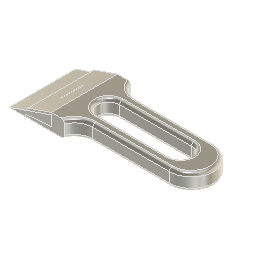
Скребок (Autodesk Fusion 360 design; units mm, degrees)
Autodesk Fusion 360 part; units mm, degrees
note: some values were not read from the file. Set by a fixed rule: which sketch regions a step uses.
sketch "Sketch1" plane through (0, 0, 0) normal (0, 0, 1) x (1, 0, 0)
  line L0 (60, -30) -> (-60, -30)
  line L1 (-60, -30) -> (-60, 30)
  line L2 (-60, 30) -> (60, 30)
  line L3 (60, -30) -> (-60, 30) construction
  line L4 (-60, -30) -> (60, 30) construction
  line L5 (-25, -20) -> (-25, 20)
  line L6 (-25, 20) -> (60, 20)
  line L7 (-25, -20) -> (60, -20)
  line L8 (-25, -20) -> (-25, -30)
  line L9 (-25, 20) -> (-25, 30)
  line L10 (-25, 10) -> (50, 10)
  line L11 (-25, -10) -> (50, -10)
  arc A0 (50, -10) -> (50, 10) centre (50, 0) ccw
  arc A1 (60, -20) -> (60, 20) centre (60, 0) ccw
  line L12 (60, 30) -> (60, 20)
  line L13 (60, -20) -> (60, -30)
  constraint horizontal L0
  constraint perpendicular L0 L1
  constraint parallel L0 L2
  constraint parallel L1 L12
  constraint coincident L3 origin
  constraint coincident L4 origin
  constraint vertical L5
  constraint perpendicular L6 L12
  constraint coincident L7.end L12
  constraint perpendicular L7 L12
  constraint perpendicular L7 L8
  constraint coincident L2 L9.end
  constraint perpendicular L2 L9
  constraint tangent L10 A0
  constraint collinear L12 L13
extrude "Extrude1" add sketch "Sketch1" along normal blind 15 contours L0 L1 L2 L5 L8 L9 | L5 L6 L7 L10 L11 A0 A1 makes body 1
sketch "Sketch2" plane through (0, -30, 0) normal (0, -1, 0) x (1, 0, 0)
  line L0 (-60, 0) -> (-25, 0)
  line L1 (-25, 0) -> (-25, 15)
  line L2 (-25, 15) -> (-60, 15)
  line L3 (-60, 15) -> (-60, 0)
  line L4 (-75.0675, 0) -> (-36.9699, 13.0336)
  line L5 (-75.0675, 0) -> (-60, 0)
  line L6 (-60, 0) -> (-60, 1.9989)
  line L7 (-60, 1.9989) -> (-36.9699, 4.0017)
  line L8 (-36.9699, 4.0017) -> (-36.9699, 13.0336)
  line L9 (-48.7521, 10.4269) -> (-47.477, 10.8632)
  line L10 (-47.477, 10.8632) -> (-47.477, 9.439)
  line L11 (-49.9999, 8.5759) -> (-48.7521, 10.4269)
  point P0 (-50.0767, 9.9738)
  constraint coincident L0.start L3.end
  constraint perpendicular L3 L5
  constraint coincident L3 L6.end
  constraint parallel L3 L8
  constraint parallel L4 L9
  constraint coincident L4 L10.end
  constraint perpendicular L0 L10
  constraint coincident P0 L9
  constraint coincident L4 L11.start
extrude "Extrude2" cut sketch "Sketch2" against normal blind 79 contours L3 L4 L5 L6 | L3 L4 L7 L8 bodies 1
sketch "Sketch3" plane through (0, -30, 0) normal (0, -1, 0) x (1, 0, 0)
  line L0 (-60, 5.1547) -> (-36.9699, 13.0336)
  line L1 (-36.9699, 13.0336) -> (-36.9699, 4.0017)
  line L2 (-36.9699, 4.0017) -> (-60, 1.9989)
  line L3 (-60, 1.9989) -> (-60, 0)
  line L4 (-60, 0) -> (-25, 0)
  line L5 (-25, 0) -> (-25, 15)
  line L6 (-25, 15) -> (-60, 15)
  line L7 (-37, 15) -> (-60, 15)
  line L8 (-60, 5.1547) -> (-60, 7.1547)
  line L9 (-60, 7.1547) -> (-60, 15)
  line L10 (-60, 7.1547) -> (-37, 15)
  dimension "d28" = 2
  constraint coincident L6 L7.start
  constraint coincident L6.end L7.end
  constraint coincident L0.start L8.start
  constraint vertical L8
  measures "d28" distance of L0.start L8.end
extrude "Extrude3" cut sketch "Sketch3" against normal blind 78 contours L6 L7 L9 L10 bodies 1
extrude "Extrude4" cut sketch "Sketch2" along normal blind -20 and the other way blind 40 contours L4 L9 L10 L11 bodies 1
fillet "Fillet1" radius 17 2 edges at (-25, 20, 7.5) (-25, -20, 7.5) on bodies 1
fillet "Fillet2" radius 3 10 edges at (-18.7276, -22.7171, 15) (25.246, -20, 15) (80, 0, 15) (25.246, 20, 15) (-18.7276, 22.7171, 15) (-18.7276, -22.7171, 0) (25.246, -20, 0) (80, 0, 0) (25.246, 20, 0) (-18.7276, 22.7171, 0) on bodies 1
extrude "Extrude5" add sketch "Sketch2" along normal blind 0 and the other way blind 60 separate body contours L3 L4 L5 L6 | L3 L4 L7 L8 makes body 2
extrude "Extrude6" add sketch "Sketch2" along normal blind -20.5 and the other way blind 39.5 contours L4 L9 L10 L11 bodies 2
fillet "Fillet3" radius 10 2 edges at (-25, 10, 7.5) (-25, -10, 7.5) on bodies 1
fillet "Fillet4" radius 3 8 edges at (17.5, -10, 15) (-25, 0, 15) (17.5, 10, 15) (60, 0, 15) (17.5, -10, 0) (-25, 0, 0) (17.5, 10, 0) (60, 0, 0) on bodies 1
chamfer "Chamfer1" distance 2 angle 45 1 edges at (-60, 0, 7.1547) on bodies 1
